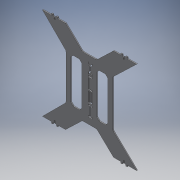
# Autodesk Inventor part: Z stage_brace
Saved by Autodesk Inventor 2019 (Build 230136000, 136)
## iProperties
Created: 2020-03-07
Part Number: Z stage_brace
Material: Generic
Document SubType Name: Modeling
Designer: Vijay
Density: 1 g/cm^3
Appearance: Default
Author: Vijay
Autodesk Inventor part; units mm, degrees
(part 1 of 2)
ref_plane "YZ Plane" through (0, 0, 0) normal (1, 0, 0) x (0, 1, 0)
ref_plane "XZ Plane" through (0, 0, 0) normal (0, 1, 0) x (-1, 0, 0)
ref_plane "XY Plane" through (0, 0, 0) normal (0, 0, 1) x (1, 0, 0)
sketch "Sketch1" plane through (0, 0, 0) normal (0, 0, 1) x (1, 0, 0)
  line L0 (428.582494, 0) -> (19.999963, 0)
  line L1 (19.999963, -400) -> (428.582494, -400)
  line L2 (328.588324, 0) -> (224.296824, -100)
  line L3 (224.296824, -100) -> (119.999963, 0)
  line L4 (328.582494, -400) -> (224.296824, -300)
  line L5 (224.296824, -300) -> (119.999963, -400)
  line L6 (224.296824, 24.036102) -> (224.296824, -493.226766) construction
  line L7 (428.582494, 0) -> (328.588324, 0)
  line L8 (119.999963, 0) -> (19.998423, 0)
  line L9 (19.999963, -400) -> (119.999963, -400)
  line L10 (328.582494, -400) -> (428.582446, -400)
  line L11 (19.998423, 0) -> (122.169678, -102.170786)
  line L12 (122.169678, -102.170786) -> (122.17075, -297.828745)
  line L13 (122.17075, -297.828745) -> (19.999963, -400)
  line L14 (428.582494, 0) -> (324.296824, -100.006079)
  line L15 (324.296824, -100.006079) -> (324.296824, -299.999951)
  line L16 (324.296824, -299.999951) -> (428.582446, -400)
  line L17 (255.584274, -70) -> (193.007766, -70)
  line L18 (255.582525, -330) -> (193.007766, -330)
  line L19 (19.999963, -400) -> (19.999963, -400)
  point P0 (0, 0)
  dimension "d1" = 100
  dimension "d2" = 100
  dimension "d3" = 100
  dimension "d4" = 104.2915
  dimension "d5" = 100
  dimension "d6" = 100
  dimension "d7" = 100
  dimension "d8" = 70
  dimension "d9" = 70
  constraints: 36 end point, 7 point on line, 4 equal length, 4 horizontal, 4 parallel, 3 perpendicular, 2 collinear, 2 vertical
  measures "d1" distance of L4.start L1.end
  measures "d2" distance of L5.end L1.start
  measures "d3" distance of L3.end L0.end
  measures "d4" distance from line of L6 L2.start
  measures "d5" distance from line of L0 L2.end
  measures "d6" distance from line of L1 L4.end
  measures "d7" distance between parallel lines of L6 L15
  measures "d8" distance between parallel lines of L0 L17
  measures "d9" distance between parallel lines of L1 L18
extrude "Extrusion1" add sketch "Sketch1" against normal blind 4 contours L14 L15 L16 L1 L4 L5 L13 L12 L11 L0 L3 L2 | L2 L3 L17 | L18 L5 L4
fillet "Fillet1" radius 10 8 edges at (324.2968, -100.0061, -2) (324.2968, -300, -2) (255.5825, -330, -2) (193.0078, -330, -2) (122.1708, -297.8287, -2) (122.1697, -102.1708, -2) (193.0078, -70, -2) (255.5843, -70, -2)
sketch "Sketch2" plane through (0, 0, -4) normal (0, 0, -1) x (-1, 0, 0)
  line L0 (-235.522226, -304.84913) -> (-235.522226, -94.876812) construction
  line L1 (-235.522226, -94.876812) -> (-217.757001, -94.876812) construction
  line L2 (-217.757001, -94.876812) -> (-217.757001, -304.84913) construction
  line L3 (-217.757001, -304.84913) -> (-235.522226, -304.84913) construction
  line L4 (-217.757, -297.116395) -> (-224.424748, -297.116395)
  line L5 (-224.424748, -297.116395) -> (-224.424748, -260.814212)
  line L6 (-224.424748, -260.814212) -> (-217.757, -260.814212)
  line L7 (-217.757, -260.814212) -> (-217.757, -255.057105)
  line L8 (-217.757, -255.057105) -> (-235.522226, -255.057105)
  line L9 (-235.522226, -255.057105) -> (-235.522226, -260.814212)
  line L10 (-235.522226, -260.814212) -> (-228.854478, -260.814212)
  line L11 (-228.854478, -260.814212) -> (-228.854478, -297.116395)
  line L12 (-228.854478, -297.116395) -> (-235.522226, -297.116395)
  line L13 (-235.522226, -297.116395) -> (-235.522226, -302.873501)
  line L14 (-235.522226, -302.873501) -> (-217.757, -302.873501)
  line L15 (-217.757, -302.873501) -> (-217.757, -297.116395)
  line L16 (-224.424748, -205.542904) -> (-228.854478, -205.542904)
  line L17 (-228.854478, -205.542904) -> (-228.854478, -245.348741)
  line L18 (-228.854478, -245.348741) -> (-229.76512, -245.348741)
  spline S0 degree 2 poles (-229.76512, -245.348741) (-230.305331, -245.348741) (-231.10793, -244.777661) (-231.10793, -244.160277) knots 0 0 0 1 2 2 2
  line L19 (-231.10793, -244.160277) -> (-231.10793, -205.4966)
  line L20 (-231.10793, -205.4966) -> (-235.522226, -205.4966)
  line L21 (-235.522226, -205.4966) -> (-235.522226, -247.170024)
  spline S1 degree 2 poles (-235.522226, -247.170024) (-235.522226, -249.238261) (-233.392251, -251.105847) (-231.555534, -251.105847) knots 0 0 0 1 2 2 2
  line L22 (-231.555534, -251.105847) -> (-221.723692, -251.105847)
  spline S2 degree 2 poles (-221.723692, -251.105847) (-219.886975, -251.105847) (-217.757, -249.238261) (-217.757, -247.170024) knots 0 0 0 1 2 2 2
  line L23 (-217.757, -247.170024) -> (-217.757, -205.4966)
  line L24 (-217.757, -205.4966) -> (-222.18673, -205.4966)
  line L25 (-222.18673, -205.4966) -> (-222.18673, -244.160277)
  spline S3 degree 2 poles (-222.18673, -244.160277) (-222.18673, -244.777661) (-222.973895, -245.348741) (-223.514106, -245.348741) knots 0 0 0 1 2 2 2
  line L26 (-223.514106, -245.348741) -> (-224.424748, -245.348741)
  line L27 (-224.424748, -245.348741) -> (-224.424748, -205.542904)
  line L28 (-235.522226, -201.545342) -> (-221.723692, -201.545342)
  spline S4 degree 2 poles (-221.723692, -201.545342) (-219.886975, -201.545342) (-217.757, -199.677755) (-217.757, -197.609519) knots 0 0 0 1 2 2 2
  line L29 (-217.757, -197.609519) -> (-217.757, -155.936094)
  line L30 (-217.757, -155.936094) -> (-222.18673, -155.936094)
  line L31 (-222.18673, -155.936094) -> (-222.18673, -194.599771)
  spline S5 degree 2 poles (-222.18673, -194.599771) (-222.18673, -195.217155) (-222.973895, -195.788236) (-223.514106, -195.788236) knots 0 0 0 1 2 2 2
  line L32 (-223.514106, -195.788236) -> (-235.522226, -195.788236)
  line L33 (-235.522226, -195.788236) -> (-235.522226, -201.545342)
  line L34 (-217.757, -146.181426) -> (-235.522226, -146.181426)
  line L35 (-235.522226, -146.181426) -> (-235.522226, -151.984836)
  line L36 (-235.522226, -151.984836) -> (-217.757, -151.984836)
  line L37 (-217.757, -151.984836) -> (-217.757, -146.181426)
  line L38 (-235.522226, -95.710279) -> (-235.522226, -103.304103)
  line L39 (-235.522226, -103.304103) -> (-228.854478, -111.422704)
  line L40 (-228.854478, -111.422704) -> (-228.854478, -127.659904)
  line L41 (-228.854478, -127.659904) -> (-235.522226, -135.778505)
  line L42 (-235.522226, -135.778505) -> (-235.522226, -143.372329)
  line L43 (-235.522226, -143.372329) -> (-226.64733, -132.768757)
  line L44 (-226.64733, -132.768757) -> (-217.757, -143.372329)
  line L45 (-217.757, -143.372329) -> (-217.757, -135.778505)
  line L46 (-217.757, -135.778505) -> (-224.424748, -127.659904)
  line L47 (-224.424748, -127.659904) -> (-224.424748, -111.422704)
  line L48 (-224.424748, -111.422704) -> (-217.757, -103.304103)
  line L49 (-217.757, -103.304103) -> (-217.757, -95.710279)
  line L50 (-217.757, -95.710279) -> (-226.64733, -106.31385)
  line L51 (-226.64733, -106.31385) -> (-235.522226, -95.710279)
  point P0 (0, 0)
  constraints: 2 other
extrude "Extrusion2" cut sketch "Sketch2" against normal blind 25.4
sketch "Sketch3" plane through (0, 0, 0) normal (0, 0, 1) x (1, 0, 0)
  line L0 (394.29103, -17.648783) -> (394.29103, 0)
  line L1 (394.29103, 0) -> (387.415198, 0)
  line L2 (387.415198, 0) -> (387.415198, 6.35)
  line L3 (387.415198, 6.35) -> (381.415186, 6.35)
  line L4 (381.415186, 6.35) -> (381.415186, 0)
  line L5 (381.415186, 0) -> (375.315187, 0)
  line L6 (375.315187, 0) -> (375.315187, -6)
  line L7 (375.315187, -6) -> (376.565186, -6)
  line L8 (376.565186, -6) -> (376.565186, -8)
  line L9 (376.565186, -8) -> (375.315187, -8)
  line L10 (375.315187, -8) -> (375.315187, -10.649999)
  line L11 (375.315187, -10.649999) -> (372.315196, -10.649999)
  line L12 (372.315196, -10.649999) -> (372.315196, -8)
  line L13 (372.315196, -8) -> (371.065197, -8)
  line L14 (371.065197, -8) -> (371.065197, -6)
  line L15 (371.065197, -6) -> (372.315196, -6)
  line L16 (372.315196, -6) -> (372.315196, 0)
  line L17 (372.315196, 0) -> (366.215197, 0)
  line L18 (366.215197, 0) -> (366.215197, 6.35)
  line L19 (366.215197, 6.35) -> (360.2152, 6.35)
  line L20 (360.2152, 6.35) -> (360.2152, 0)
  line L21 (360.2152, 0) -> (353.339353, 0)
  line L22 (353.339353, 0) -> (353.339353, -17.648783)
  line L23 (353.339353, -17.648783) -> (394.29103, -17.648783)
  line L24 (353.340387, -382.350485) -> (353.340487, -399.999268)
  line L25 (353.340487, -399.999268) -> (360.216319, -399.999229)
  line L26 (360.216319, -399.999229) -> (360.216355, -406.349229)
  line L27 (360.216355, -406.349229) -> (366.216367, -406.349195)
  line L28 (366.216367, -406.349195) -> (366.216331, -399.999195)
  line L29 (366.216331, -399.999195) -> (372.31633, -399.999161)
  line L30 (372.31633, -399.999161) -> (372.316296, -393.999161)
  line L31 (372.316296, -393.999161) -> (371.066297, -393.999168)
  line L32 (371.066297, -393.999168) -> (371.066286, -391.999167)
  line L33 (371.066286, -391.999167) -> (372.316284, -391.99916)
  line L34 (372.316284, -391.99916) -> (372.316269, -389.349161)
  line L35 (372.316269, -389.349161) -> (375.316261, -389.349144)
  line L36 (375.316261, -389.349144) -> (375.316276, -391.999143)
  line L37 (375.316276, -391.999143) -> (376.566274, -391.999136)
  line L38 (376.566274, -391.999136) -> (376.566286, -393.999137)
  line L39 (376.566286, -393.999137) -> (375.316287, -393.999144)
  line L40 (375.316287, -393.999144) -> (375.316321, -399.999144)
  line L41 (375.316321, -399.999144) -> (381.41632, -399.999109)
  line L42 (381.41632, -399.999109) -> (381.416356, -406.349109)
  line L43 (381.416356, -406.349109) -> (387.416353, -406.349075)
  line L44 (387.416353, -406.349075) -> (387.416317, -399.999075)
  line L45 (387.416317, -399.999075) -> (394.292164, -399.999036)
  line L46 (394.292164, -399.999036) -> (394.292064, -382.350253)
  line L47 (394.292064, -382.350253) -> (353.340387, -382.350485)
  line L48 (93.121147, -17.649526) -> (93.121047, -0.000743)
  line L49 (93.121047, -0.000743) -> (86.245215, -0.000782)
  line L50 (86.245215, -0.000782) -> (86.245179, 6.349218)
  line L51 (86.245179, 6.349218) -> (80.245166, 6.349184)
  line L52 (80.245166, 6.349184) -> (80.245202, -0.000816)
  line L53 (80.245202, -0.000816) -> (74.145203, -0.000851)
  line L54 (74.145203, -0.000851) -> (74.145237, -6.000851)
  line L55 (74.145237, -6.000851) -> (75.395236, -6.000844)
  line L56 (75.395236, -6.000844) -> (75.395248, -8.000844)
  line L57 (75.395248, -8.000844) -> (74.145249, -8.000851)
  line L58 (74.145249, -8.000851) -> (74.145264, -10.65085)
  line L59 (74.145264, -10.65085) -> (71.145273, -10.650867)
  line L60 (71.145273, -10.650867) -> (71.145258, -8.000868)
  line L61 (71.145258, -8.000868) -> (69.895259, -8.000875)
  line L62 (69.895259, -8.000875) -> (69.895247, -6.000875)
  line L63 (69.895247, -6.000875) -> (71.145246, -6.000868)
  line L64 (71.145246, -6.000868) -> (71.145212, -0.000868)
  line L65 (71.145212, -0.000868) -> (65.045213, -0.000902)
  line L66 (65.045213, -0.000902) -> (65.045177, 6.349097)
  line L67 (65.045177, 6.349097) -> (59.04518, 6.349063)
  line L68 (59.04518, 6.349063) -> (59.045216, -0.000936)
  line L69 (59.045216, -0.000936) -> (52.169369, -0.000975)
  line L70 (52.169369, -0.000975) -> (52.169469, -17.649759)
  line L71 (52.169469, -17.649759) -> (93.121147, -17.649526)
  line L72 (52.171537, -382.352192) -> (52.171637, -400.000976)
  line L73 (52.171637, -400.000976) -> (59.047469, -400.000937)
  line L74 (59.047469, -400.000937) -> (59.047505, -406.350936)
  line L75 (59.047505, -406.350936) -> (65.047517, -406.350902)
  line L76 (65.047517, -406.350902) -> (65.047481, -400.000903)
  line L77 (65.047481, -400.000903) -> (71.14748, -400.000868)
  line L78 (71.14748, -400.000868) -> (71.147446, -394.000868)
  line L79 (71.147446, -394.000868) -> (69.897447, -394.000875)
  line L80 (69.897447, -394.000875) -> (69.897436, -392.000875)
  line L81 (69.897436, -392.000875) -> (71.147434, -392.000868)
  line L82 (71.147434, -392.000868) -> (71.147419, -389.350868)
  line L83 (71.147419, -389.350868) -> (74.14741, -389.350851)
  line L84 (74.14741, -389.350851) -> (74.147426, -392.000851)
  line L85 (74.147426, -392.000851) -> (75.397424, -392.000843)
  line L86 (75.397424, -392.000843) -> (75.397436, -394.000844)
  line L87 (75.397436, -394.000844) -> (74.147437, -394.000851)
  line L88 (74.147437, -394.000851) -> (74.147471, -400.000851)
  line L89 (74.147471, -400.000851) -> (80.24747, -400.000816)
  line L90 (80.24747, -400.000816) -> (80.247506, -406.350816)
  line L91 (80.247506, -406.350816) -> (86.247503, -406.350782)
  line L92 (86.247503, -406.350782) -> (86.247467, -400.000782)
  line L93 (86.247467, -400.000782) -> (93.123314, -400.000743)
  line L94 (93.123314, -400.000743) -> (93.123214, -382.35196)
  line L95 (93.123214, -382.35196) -> (52.171537, -382.352192)
  point P0 (0, 0)
extrude "Extrusion3" add sketch "Sketch3" against normal up to surface (4 mm away)
sketch "Sketch4" plane through (0, 0, 0) normal (0, 0, 1) x (1, 0, 0)
  line L0 (394.29103, -17.648783) -> (394.29103, 0)
  line L1 (394.29103, 0) -> (387.415198, 0)
  line L2 (387.415198, 0) -> (387.415198, 6.35)
  line L3 (387.415198, 6.35) -> (381.415186, 6.35)
  line L4 (381.415186, 6.35) -> (381.415186, 0)
  line L5 (381.415186, 0) -> (375.315187, 0)
  line L6 (375.315187, 0) -> (375.315187, -6)
  line L7 (375.315187, -6) -> (376.565186, -6)
  line L8 (376.565186, -6) -> (376.565186, -8)
  line L9 (376.565186, -8) -> (375.315187, -8)
  line L10 (375.315187, -8) -> (375.315187, -10.649999)
  line L11 (375.315187, -10.649999) -> (372.315196, -10.649999)
  line L12 (372.315196, -10.649999) -> (372.315196, -8)
  line L13 (372.315196, -8) -> (371.065197, -8)
  line L14 (371.065197, -8) -> (371.065197, -6)
  line L15 (371.065197, -6) -> (372.315196, -6)
  line L16 (372.315196, -6) -> (372.315196, 0)
  line L17 (372.315196, 0) -> (366.215197, 0)
  line L18 (366.215197, 0) -> (366.215197, 6.35)
  line L19 (366.215197, 6.35) -> (360.2152, 6.35)
  line L20 (360.2152, 6.35) -> (360.2152, 0)
  line L21 (360.2152, 0) -> (353.339353, 0)
  line L22 (353.339353, 0) -> (353.339353, -17.648783)
  line L23 (353.339353, -17.648783) -> (394.29103, -17.648783)
  line L24 (353.340387, -382.350485) -> (353.340487, -399.999268)
  line L25 (353.340487, -399.999268) -> (360.216319, -399.999229)
  line L26 (360.216319, -399.999229) -> (360.216355, -406.349229)
  line L27 (360.216355, -406.349229) -> (366.216367, -406.349195)
  line L28 (366.216367, -406.349195) -> (366.216331, -400)
  line L29 (366.216331, -399.999195) -> (372.31633, -399.999161)
  line L30 (372.31633, -399.999161) -> (372.316296, -393.999161)
  line L31 (372.316296, -393.999161) -> (371.066297, -393.999168)
  line L32 (371.066297, -393.999168) -> (371.066286, -391.999167)
  line L33 (371.066286, -391.999167) -> (372.316284, -391.99916)
  line L34 (372.316284, -391.99916) -> (372.316269, -389.349161)
  line L35 (372.316269, -389.349161) -> (375.316261, -389.349144)
  line L36 (375.316261, -389.349144) -> (375.316276, -391.999143)
  line L37 (375.316276, -391.999143) -> (376.566274, -391.999136)
  line L38 (376.566274, -391.999136) -> (376.566286, -393.999137)
  line L39 (376.566286, -393.999137) -> (375.316287, -393.999144)
  line L40 (375.316287, -393.999144) -> (375.316321, -399.999144)
  line L41 (375.316321, -399.999144) -> (381.41632, -399.999109)
  line L42 (381.41632, -400) -> (381.416356, -406.349109)
  line L43 (381.416356, -406.349109) -> (387.416353, -406.349075)
  line L44 (387.416353, -406.349075) -> (387.416317, -399.999075)
  line L45 (387.416317, -399.999075) -> (394.292164, -399.999036)
  line L46 (394.292164, -399.999036) -> (394.292064, -382.350253)
  line L47 (394.292064, -382.350253) -> (353.340387, -382.350485)
  line L48 (52.171537, -382.352192) -> (52.171637, -400.000976)
  line L49 (52.171637, -400.000976) -> (59.047469, -400.000937)
  line L50 (59.047469, -400.000937) -> (59.047505, -406.350936)
  line L51 (59.047505, -406.350936) -> (65.047517, -406.350902)
  line L52 (65.047517, -406.350902) -> (65.047481, -400.000159)
  line L53 (93.123314, -400.000743) -> (71.14748, -400.000868)
  line L54 (71.14748, -400.000868) -> (71.147446, -394.000868)
  line L55 (71.147446, -394.000868) -> (69.897447, -394.000875)
  line L56 (69.897447, -394.000875) -> (69.897436, -392.000875)
  line L57 (69.897436, -392.000875) -> (71.147434, -392.000868)
  line L58 (71.147434, -392.000868) -> (71.147419, -389.350868)
  line L59 (71.147419, -389.350868) -> (74.14741, -389.350851)
  line L60 (74.14741, -389.350851) -> (74.147426, -392.000851)
  line L61 (74.147426, -392.000851) -> (75.397424, -392.000843)
  line L62 (75.397424, -392.000843) -> (75.397436, -394.000844)
  line L63 (75.397436, -394.000844) -> (74.147437, -394.000851)
  line L64 (74.147437, -394.000851) -> (74.147471, -400.000851)
  line L65 (74.147471, -400.000851) -> (119.999963, -400.000591)
  line L66 (80.24747, -400.000225) -> (80.247506, -406.350816)
  line L67 (80.247506, -406.350816) -> (86.247503, -406.350782)
  line L68 (86.247503, -406.350782) -> (86.247467, -400.000782)
  line L69 (86.247467, -400.000782) -> (93.123314, -400.000743)
  line L70 (93.123314, -400.000743) -> (93.123214, -382.35196)
  line L71 (93.123214, -382.35196) -> (52.171537, -382.352192)
  line L72 (93.121147, -17.649526) -> (93.121047, -0.000743)
  line L73 (93.121047, -0.000743) -> (86.245215, -0.000782)
  line L74 (86.245215, -0.000782) -> (86.245179, 6.349218)
  line L75 (86.245179, 6.349218) -> (80.245166, 6.349184)
  line L76 (80.245166, 6.349184) -> (80.245202, 0)
  line L77 (80.245202, -0.000816) -> (74.145203, -0.000851)
  line L78 (74.145203, -0.000851) -> (74.145237, -6.000851)
  line L79 (74.145237, -6.000851) -> (75.395236, -6.000844)
  line L80 (75.395236, -6.000844) -> (75.395248, -8.000844)
  line L81 (75.395248, -8.000844) -> (74.145249, -8.000851)
  line L82 (74.145249, -8.000851) -> (74.145264, -10.65085)
  line L83 (74.145264, -10.65085) -> (71.145273, -10.650867)
  line L84 (71.145273, -10.650867) -> (71.145258, -8.000868)
  line L85 (71.145258, -8.000868) -> (69.895259, -8.000875)
  line L86 (69.895259, -8.000875) -> (69.895247, -6.000875)
  line L87 (69.895247, -6.000875) -> (71.145246, -6.000868)
  line L88 (71.145246, -6.000868) -> (71.145212, -0.000868)
  line L89 (71.145212, -0.000868) -> (65.045213, -0.000902)
  line L90 (65.045213, 0) -> (65.045177, 6.349097)
  line L91 (65.045177, 6.349097) -> (59.04518, 6.349063)
  line L92 (59.04518, 6.349063) -> (59.045216, -0.000936)
  line L93 (59.045216, -0.000936) -> (52.169369, -0.000975)
  line L94 (52.169369, -0.000975) -> (52.169469, -17.649759)
  line L95 (52.169469, -17.649759) -> (93.121147, -17.649526)
  line L96 (375.315187, 0) -> (372.315196, 0)
  line L97 (375.316321, -400) -> (372.31633, -400)
  line L98 (366.216331, -400) -> (381.41632, -400)
  line L99 (74.147471, -400) -> (71.14748, -400)
  line L100 (119.999963, -400) -> (93.123314, -400)
  line L101 (74.145203, 0) -> (71.145212, 0)
  line L102 (65.045213, 0) -> (80.245202, 0)
  point P0 (0, 0)
  point P1 (93.123314, -400)
  point P2 (119.999963, -400)
  constraints: 8 end point, 3 horizontal, 1 perpendicular, 3 other
extrude "Extrusion4" cut sketch "Sketch4" against normal blind 25.4 contours L6 L7 L8 L9 L10 L11 L12 L13 L14 L15 L16 L96 | L30 L31 L32 L33 L34 L35 L36 L37 L38 L39 L40 L97 | L53 L54 L55 L56 L57 L58 L59 L60 L61 L62 L63 L64 | L78 L79 L80 L81 L82 L83 L84 L85 L86 L87 L88 L101
sketch "Sketch5" plane through (0, 0, -4) normal (0, 0, -1) x (-1, 0, 0)
  line L0 (-228.854478, -111.422704) -> (-235.522226, -103.304103)
  line L1 (-235.522226, -103.304103) -> (-235.522226, -95.710279)
  line L2 (-235.522226, -95.710279) -> (-226.64733, -106.31385)
  line L3 (-226.64733, -106.31385) -> (-217.757, -95.710279)
  line L4 (-217.757, -95.710279) -> (-217.757, -103.304103)
  line L5 (-217.757, -103.304103) -> (-224.424748, -111.422704)
  line L6 (-224.424748, -111.422704) -> (-224.424748, -127.659904)
  line L7 (-224.424748, -127.659904) -> (-217.757, -135.778505)
  line L8 (-217.757, -135.778505) -> (-217.757, -143.372329)
  line L9 (-217.757, -143.372329) -> (-226.64733, -132.768757)
  line L10 (-226.64733, -132.768757) -> (-235.522226, -143.372329)
  line L11 (-235.522226, -143.372329) -> (-235.522226, -135.778505)
  line L12 (-235.522226, -135.778505) -> (-228.854478, -127.659904)
  line L13 (-228.854478, -127.659904) -> (-228.854478, -111.422704)
  line L14 (-221.723692, -201.545342) -> (-235.522226, -201.545342)
  line L15 (-235.522226, -201.545342) -> (-235.522226, -195.788236)
  line L16 (-235.522226, -195.788236) -> (-223.514106, -195.788236)
  line L17 (-222.18673, -194.599771) -> (-222.18673, -155.936094)
  line L18 (-222.18673, -155.936094) -> (-217.757, -155.936094)
  line L19 (-217.757, -155.936094) -> (-217.757, -197.609519)
  line L20 (-224.424748, -260.814212) -> (-224.424748, -297.116395)
  line L21 (-224.424748, -297.116395) -> (-217.757, -297.116395)
  line L22 (-217.757, -297.116395) -> (-217.757, -302.873501)
  line L23 (-217.757, -302.873501) -> (-235.522226, -302.873501)
  line L24 (-235.522226, -302.873501) -> (-235.522226, -297.116395)
  line L25 (-235.522226, -297.116395) -> (-228.854478, -297.116395)
  line L26 (-228.854478, -297.116395) -> (-228.854478, -260.814212)
  line L27 (-228.854478, -260.814212) -> (-235.522226, -260.814212)
  line L28 (-235.522226, -260.814212) -> (-235.522226, -255.057105)
  line L29 (-235.522226, -255.057105) -> (-217.757, -255.057105)
  line L30 (-217.757, -255.057105) -> (-217.757, -260.814212)
  line L31 (-217.757, -260.814212) -> (-224.424748, -260.814212)
  line L32 (-228.854478, -245.348741) -> (-228.854478, -205.542904)
  line L33 (-228.854478, -205.542904) -> (-224.424748, -205.542904)
  line L34 (-224.424748, -205.542904) -> (-224.424748, -245.348741)
  line L35 (-224.424748, -245.348741) -> (-223.514106, -245.348741)
  line L36 (-222.18673, -244.160277) -> (-222.18673, -205.4966)
  line L37 (-222.18673, -205.4966) -> (-217.757, -205.4966)
  line L38 (-217.757, -205.4966) -> (-217.757, -247.170024)
  line L39 (-221.723692, -251.105847) -> (-231.555534, -251.105847)
  line L40 (-235.522226, -247.170024) -> (-235.522226, -205.4966)
  line L41 (-235.522226, -205.4966) -> (-231.10793, -205.4966)
  line L42 (-231.10793, -205.4966) -> (-231.10793, -244.160277)
  line L43 (-229.76512, -245.348741) -> (-228.854478, -245.348741)
  line L44 (-235.522226, -151.984836) -> (-235.522226, -146.181426)
  line L45 (-235.522226, -146.181426) -> (-217.757, -146.181426)
  line L46 (-217.757, -146.181426) -> (-217.757, -151.984836)
  line L47 (-217.757, -151.984836) -> (-235.522226, -151.984836)
  line L48 (-71.145212, -0.000868) -> (-71.145246, -6.000868)
  line L49 (-71.145246, -6.000868) -> (-69.895247, -6.000875)
  line L50 (-69.895247, -6.000875) -> (-69.895259, -8.000875)
  line L51 (-69.895259, -8.000875) -> (-71.145258, -8.000868)
  line L52 (-71.145258, -8.000868) -> (-71.145273, -10.650867)
  line L53 (-71.145273, -10.650867) -> (-74.145264, -10.65085)
  line L54 (-74.145264, -10.65085) -> (-74.145249, -8.000851)
  line L55 (-74.145249, -8.000851) -> (-75.395248, -8.000844)
  line L56 (-75.395248, -8.000844) -> (-75.395236, -6.000844)
  line L57 (-75.395236, -6.000844) -> (-74.145237, -6.000851)
  line L58 (-74.145237, -6.000851) -> (-74.145203, -0.000851)
  line L59 (-74.145203, -0.000851) -> (-71.145212, -0.000868)
  line L60 (-375.316321, -399.999144) -> (-375.316287, -393.999144)
  line L61 (-375.316287, -393.999144) -> (-376.566286, -393.999137)
  line L62 (-376.566286, -393.999137) -> (-376.566274, -391.999136)
  line L63 (-376.566274, -391.999136) -> (-375.316276, -391.999143)
  line L64 (-375.316276, -391.999143) -> (-375.316261, -389.349144)
  line L65 (-375.316261, -389.349144) -> (-372.316269, -389.349161)
  line L66 (-372.316269, -389.349161) -> (-372.316284, -391.99916)
  line L67 (-372.316284, -391.99916) -> (-371.066286, -391.999167)
  line L68 (-371.066286, -391.999167) -> (-371.066297, -393.999168)
  line L69 (-371.066297, -393.999168) -> (-372.316296, -393.999161)
  line L70 (-372.316296, -393.999161) -> (-372.31633, -399.999161)
  line L71 (-372.31633, -399.999161) -> (-375.316321, -399.999144)
  line L72 (-74.147471, -400.000851) -> (-74.147437, -394.000851)
  line L73 (-74.147437, -394.000851) -> (-75.397436, -394.000844)
  line L74 (-75.397436, -394.000844) -> (-75.397424, -392.000843)
  line L75 (-75.397424, -392.000843) -> (-74.147426, -392.000851)
  line L76 (-74.147426, -392.000851) -> (-74.14741, -389.350851)
  line L77 (-74.14741, -389.350851) -> (-71.147419, -389.350868)
  line L78 (-71.147419, -389.350868) -> (-71.147434, -392.000868)
  line L79 (-71.147434, -392.000868) -> (-69.897436, -392.000875)
  line L80 (-69.897436, -392.000875) -> (-69.897447, -394.000875)
  line L81 (-69.897447, -394.000875) -> (-71.147446, -394.000868)
  line L82 (-71.14748, -400.000868) -> (-71.147446, -394.000868)
  line L83 (-65.047481, -400.000903) -> (-71.14748, -400.000868)
  line L84 (-65.047517, -406.350902) -> (-65.047481, -400.000903)
  line L85 (-59.047505, -406.350936) -> (-65.047517, -406.350902)
  line L86 (-59.047469, -400.000937) -> (-59.047505, -406.350936)
  line L87 (-52.171637, -400.000976) -> (-59.047469, -400.000937)
  line L88 (-52.171637, -400) -> (-52.171637, -400.000976)
  line L89 (-52.171637, -400) -> (-19.999963, -400)
  line L90 (-19.999963, -400) -> (-119.241811, -300.757697)
  arc A0 (-122.170727, -293.68659) -> (-119.241811, -300.757697) centre (-112.170727, -293.686645) ccw
  line L91 (-122.170727, -293.68659) -> (-122.1697, -106.312903)
  arc A1 (-119.240752, -99.241874) -> (-122.1697, -106.312903) centre (-112.1697, -106.312958) ccw
  line L92 (-119.240752, -99.241874) -> (-19.998423, 0)
  line L93 (-19.998423, 0) -> (-59.045216, 0)
  line L94 (-59.04518, 6.349063) -> (-59.045216, 0)
  line L95 (-65.045177, 6.349097) -> (-59.04518, 6.349063)
  line L96 (-65.045213, 0) -> (-65.045177, 6.349097)
  line L97 (-65.045213, 0) -> (-80.245202, 0)
  line L98 (-80.245166, 6.349184) -> (-80.245202, 0)
  line L99 (-86.245179, 6.349218) -> (-80.245166, 6.349184)
  line L100 (-86.245215, 0) -> (-86.245179, 6.349218)
  line L101 (-86.245215, 0) -> (-119.999963, 0)
  line L102 (-119.999963, 0) -> (-190.106428, -67.218193)
  arc A2 (-197.027244, -70) -> (-190.106428, -67.218193) centre (-197.027244, -60) ccw
  line L103 (-197.027244, -70) -> (-251.564646, -70)
  arc A3 (-258.485647, -67.218015) -> (-251.564646, -70) centre (-251.564646, -60) ccw
  line L104 (-258.485647, -67.218015) -> (-328.588324, 0)
  line L105 (-328.588324, 0) -> (-360.2152, 0)
  line L106 (-360.2152, 6.35) -> (-360.2152, 0)
  line L107 (-366.215197, 6.35) -> (-360.2152, 6.35)
  line L108 (-366.215197, 0) -> (-366.215197, 6.35)
  line L109 (-366.215197, 0) -> (-372.315196, 0)
  line L110 (-372.315196, 0) -> (-372.315196, -6)
  line L111 (-372.315196, -6) -> (-371.065197, -6)
  line L112 (-371.065197, -6) -> (-371.065197, -8)
  line L113 (-371.065197, -8) -> (-372.315196, -8)
  line L114 (-372.315196, -8) -> (-372.315196, -10.649999)
  line L115 (-372.315196, -10.649999) -> (-375.315187, -10.649999)
  line L116 (-375.315187, -10.649999) -> (-375.315187, -8)
  line L117 (-375.315187, -8) -> (-376.565186, -8)
  line L118 (-376.565186, -8) -> (-376.565186, -6)
  line L119 (-376.565186, -6) -> (-375.315187, -6)
  line L120 (-375.315187, -6) -> (-375.315187, 0)
  line L121 (-375.315187, 0) -> (-381.415186, 0)
  line L122 (-381.415186, 6.35) -> (-381.415186, 0)
  line L123 (-387.415198, 6.35) -> (-381.415186, 6.35)
  line L124 (-387.415198, 0) -> (-387.415198, 6.35)
  line L125 (-387.415198, 0) -> (-428.582494, 0)
  line L126 (-428.582494, 0) -> (-327.375402, -97.053837)
  arc A4 (-324.296824, -104.271449) -> (-327.375402, -97.053837) centre (-334.296824, -104.271449) ccw
  line L127 (-324.296824, -104.271449) -> (-324.296824, -295.734404)
  arc A5 (-327.375618, -302.952223) -> (-324.296824, -295.734404) centre (-334.296824, -295.734404) ccw
  line L128 (-327.375618, -302.952223) -> (-428.582446, -400)
  line L129 (-428.582446, -400) -> (-387.416317, -400)
  line L130 (-387.416353, -406.349075) -> (-387.416317, -400)
  line L131 (-381.416356, -406.349109) -> (-387.416353, -406.349075)
  line L132 (-381.41632, -400) -> (-381.416356, -406.349109)
  line L133 (-381.41632, -400) -> (-366.216331, -400)
  line L134 (-366.216367, -406.349195) -> (-366.216331, -400)
  line L135 (-360.216355, -406.349229) -> (-366.216367, -406.349195)
  line L136 (-360.216319, -400) -> (-360.216355, -406.349229)
  line L137 (-360.216319, -400) -> (-328.582494, -400)
  line L138 (-328.582494, -400) -> (-258.483937, -332.782178)
  arc A6 (-251.562735, -330) -> (-258.483937, -332.782178) centre (-251.562735, -340) ccw
  line L139 (-251.562735, -330) -> (-197.027244, -330)
  arc A7 (-190.106428, -332.781807) -> (-197.027244, -330) centre (-197.027244, -340) ccw
  line L140 (-190.106428, -332.781807) -> (-119.999963, -400)
  line L141 (-119.999963, -400) -> (-93.123314, -400)
  line L142 (-93.123314, -400.000743) -> (-93.123314, -400)
  line L143 (-86.247467, -400.000782) -> (-93.123314, -400.000743)
  line L144 (-86.247503, -406.350782) -> (-86.247467, -400.000782)
  line L145 (-80.247506, -406.350816) -> (-86.247503, -406.350782)
  line L146 (-80.24747, -400.000816) -> (-80.247506, -406.350816)
  line L147 (-74.147471, -400.000851) -> (-80.24747, -400.000816)
  line L148 (-255.300194, -104.271449) -> (-304.296824, -104.271449)
  line L149 (-304.296824, -104.271449) -> (-304.296824, -295.734404)
  line L150 (-304.296824, -295.734404) -> (-255.300194, -295.734404)
  line L151 (-255.300194, -295.734404) -> (-255.300194, -104.271449)
  line L152 (-255.300194, -104.271449) -> (-304.296824, -295.734404) construction
  line L153 (-304.296824, -104.271449) -> (-255.300194, -295.734404) construction
  line L154 (-191.167357, -104.271449) -> (-142.170727, -104.271449)
  line L155 (-142.170727, -104.271449) -> (-142.170727, -295.734404)
  line L156 (-142.170727, -295.734404) -> (-191.167357, -295.734404)
  line L157 (-191.167357, -295.734404) -> (-191.167357, -104.271449)
  line L158 (-191.167357, -104.271449) -> (-142.170727, -295.734404) construction
  line L159 (-142.170727, -104.271449) -> (-191.167357, -295.734404) construction
  point P0 (0, 0)
  point P1 (-279.798509, -200.002927)
  point P2 (-166.669042, -200.002927)
  dimension "d19" = 20
  dimension "d20" = 20
  constraints: 24 end point, 4 midpoint, 4 parallel, 3 collinear, 2 horizontal, 2 perpendicular, 2 point on line, 6 other
  measures "d19" distance between parallel lines of L149 L127
  measures "d20" horizontal distance of L91.start L155.end
extrude "Extrusion5" cut sketch "Sketch5" against normal through all contours L151 L150 L149 L148 | L154 L155 L156 L157
chamfer "Chamfer1" distance 11.1125 angle 45 8 edges at (304.2968, -295.7344, -2) (255.3002, -295.7344, -2) (255.3002, -104.2714, -2) (304.2968, -104.2714, -2) (191.1674, -295.7344, -2) (142.1707, -295.7344, -2) (142.1707, -104.2714, -2) (191.1674, -104.2714, -2)
sketch "Sketch6" plane through (0, 0, 0) normal (0, 0, 1) x (1, 0, 0)
  line L0 (304.296824, -115.383949) -> (304.296824, -284.621904)
  line L1 (293.184324, -295.734404) -> (304.296824, -284.621904)
  line L2 (293.184324, -295.734404) -> (266.412694, -295.734404)
  line L3 (255.300194, -284.621904) -> (266.412694, -295.734404)
  line L4 (255.300194, -284.621904) -> (255.300194, -115.383949)
  line L5 (266.412694, -104.271449) -> (255.300194, -115.383949)
  line L6 (266.412694, -104.271449) -> (293.184324, -104.271449)
  line L7 (304.296824, -115.383949) -> (293.184324, -104.271449)
  line L8 (191.167357, -115.383949) -> (191.167357, -284.621904)
  line L9 (180.054857, -295.734404) -> (191.167357, -284.621904)
  line L10 (180.054857, -295.734404) -> (153.283227, -295.734404)
  line L11 (142.170727, -284.621904) -> (153.283227, -295.734404)
  line L12 (142.170727, -284.621904) -> (142.170727, -115.383949)
  line L13 (153.283227, -104.271449) -> (142.170727, -115.383949)
  line L14 (153.283227, -104.271449) -> (180.054857, -104.271449)
  line L15 (191.167357, -115.383949) -> (180.054857, -104.271449)
  line L16 (74.147437, -394.000851) -> (74.147471, -400.000851)
  line L17 (74.147471, -400.000851) -> (80.24747, -400.000816)
  line L18 (80.24747, -400.000816) -> (80.247506, -406.350816)
  line L19 (80.247506, -406.350816) -> (86.247503, -406.350782)
  line L20 (86.247503, -406.350782) -> (86.247467, -400.000782)
  line L21 (86.247467, -400.000782) -> (93.123314, -400.000743)
  line L22 (93.123314, -400.000743) -> (93.123314, -400)
  line L23 (93.123314, -400) -> (119.999963, -400)
  line L24 (119.999963, -400) -> (190.106428, -332.781807)
  arc A0 (197.027244, -330) -> (190.106428, -332.781807) centre (197.027244, -340) ccw
  line L25 (197.027244, -330) -> (251.562735, -330)
  arc A1 (258.483937, -332.782178) -> (251.562735, -330) centre (251.562735, -340) ccw
  line L26 (258.483937, -332.782178) -> (328.582494, -400)
  line L27 (328.582494, -400) -> (360.216319, -400)
  line L28 (360.216319, -400) -> (360.216355, -406.349229)
  line L29 (360.216355, -406.349229) -> (366.216367, -406.349195)
  line L30 (366.216367, -406.349195) -> (366.216331, -400)
  line L31 (366.216331, -400) -> (381.41632, -400)
  line L32 (381.41632, -400) -> (381.416356, -406.349109)
  line L33 (381.416356, -406.349109) -> (387.416353, -406.349075)
  line L34 (387.416353, -406.349075) -> (387.416317, -400)
  line L35 (387.416317, -400) -> (428.582446, -400)
  line L36 (428.582446, -400) -> (327.375618, -302.952223)
  arc A2 (324.296824, -295.734404) -> (327.375618, -302.952223) centre (334.296824, -295.734404) ccw
  line L37 (324.296824, -295.734404) -> (324.296824, -104.271449)
  arc A3 (327.375402, -97.053837) -> (324.296824, -104.271449) centre (334.296824, -104.271449) ccw
  line L38 (327.375402, -97.053837) -> (428.582494, 0)
  line L39 (428.582494, 0) -> (387.415198, 0)
  line L40 (387.415198, 0) -> (387.415198, 6.35)
  line L41 (387.415198, 6.35) -> (381.415186, 6.35)
  line L42 (381.415186, 6.35) -> (381.415186, 0)
  line L43 (381.415186, 0) -> (375.315187, 0)
  line L44 (375.315187, 0) -> (375.315187, -6)
  line L45 (375.315187, -6) -> (376.565186, -6)
  line L46 (376.565186, -6) -> (376.565186, -8)
  line L47 (376.565186, -8) -> (375.315187, -8)
  line L48 (375.315187, -8) -> (375.315187, -10.649999)
  line L49 (375.315187, -10.649999) -> (372.315196, -10.649999)
  line L50 (372.315196, -10.649999) -> (372.315196, -8)
  line L51 (372.315196, -8) -> (371.065197, -8)
  line L52 (371.065197, -8) -> (371.065197, -6)
  line L53 (371.065197, -6) -> (372.315196, -6)
  line L54 (372.315196, -6) -> (372.315196, 0)
  line L55 (372.315196, 0) -> (366.215197, 0)
  line L56 (366.215197, 0) -> (366.215197, 6.35)
  line L57 (366.215197, 6.35) -> (360.2152, 6.35)
  line L58 (360.2152, 6.35) -> (360.2152, 0)
  line L59 (360.2152, 0) -> (328.588324, 0)
  line L60 (328.588324, 0) -> (258.485647, -67.218015)
  arc A4 (251.564646, -70) -> (258.485647, -67.218015) centre (251.564646, -60) ccw
  line L61 (251.564646, -70) -> (197.027244, -70)
  arc A5 (190.106428, -67.218193) -> (197.027244, -70) centre (197.027244, -60) ccw
  line L62 (190.106428, -67.218193) -> (119.999963, 0)
  line L63 (119.999963, 0) -> (86.245215, 0)
  line L64 (86.245215, 0) -> (86.245179, 6.349218)
  line L65 (86.245179, 6.349218) -> (80.245166, 6.349184)
  line L66 (80.245166, 6.349184) -> (80.245202, 0)
  line L67 (80.245202, 0) -> (65.045213, 0)
  line L68 (65.045213, 0) -> (65.045177, 6.349097)
  line L69 (65.045177, 6.349097) -> (59.04518, 6.349063)
  line L70 (59.04518, 6.349063) -> (59.045216, 0)
  line L71 (59.045216, 0) -> (19.998423, 0)
  line L72 (19.998423, 0) -> (119.240752, -99.241874)
  arc A6 (122.1697, -106.312903) -> (119.240752, -99.241874) centre (112.1697, -106.312958) ccw
  line L73 (122.1697, -106.312903) -> (122.170727, -293.68659)
  arc A7 (119.241811, -300.757697) -> (122.170727, -293.68659) centre (112.170727, -293.686645) ccw
  line L74 (119.241811, -300.757697) -> (19.999963, -400)
  line L75 (19.999963, -400) -> (52.171637, -400)
  line L76 (52.171637, -400) -> (52.171637, -400.000976)
  line L77 (52.171637, -400.000976) -> (59.047469, -400.000937)
  line L78 (59.047469, -400.000937) -> (59.047505, -406.350936)
  line L79 (59.047505, -406.350936) -> (65.047517, -406.350902)
  line L80 (65.047517, -406.350902) -> (65.047481, -400.000903)
  line L81 (65.047481, -400.000903) -> (71.14748, -400.000868)
  line L82 (71.14748, -400.000868) -> (71.147446, -394.000868)
  line L83 (71.147446, -394.000868) -> (69.897447, -394.000875)
  line L84 (69.897447, -394.000875) -> (69.897436, -392.000875)
  line L85 (69.897436, -392.000875) -> (71.147434, -392.000868)
  line L86 (71.147434, -392.000868) -> (71.147419, -389.350868)
  line L87 (71.147419, -389.350868) -> (74.14741, -389.350851)
  line L88 (74.14741, -389.350851) -> (74.147426, -392.000851)
  line L89 (74.147426, -392.000851) -> (75.397424, -392.000843)
  line L90 (75.397424, -392.000843) -> (75.397436, -394.000844)
  line L91 (75.397436, -394.000844) -> (74.147437, -394.000851)
  line L92 (375.316287, -393.999144) -> (375.316321, -399.999144)
  line L93 (375.316321, -399.999144) -> (372.31633, -399.999161)
  line L94 (372.31633, -399.999161) -> (372.316296, -393.999161)
  line L95 (372.316296, -393.999161) -> (371.066297, -393.999168)
  line L96 (371.066297, -393.999168) -> (371.066286, -391.999167)
  line L97 (371.066286, -391.999167) -> (372.316284, -391.99916)
  line L98 (372.316284, -391.99916) -> (372.316269, -389.349161)
  line L99 (372.316269, -389.349161) -> (375.316261, -389.349144)
  line L100 (375.316261, -389.349144) -> (375.316276, -391.999143)
  line L101 (375.316276, -391.999143) -> (376.566274, -391.999136)
  line L102 (376.566274, -391.999136) -> (376.566286, -393.999137)
  line L103 (376.566286, -393.999137) -> (375.316287, -393.999144)
  line L104 (71.145246, -6.000868) -> (71.145212, -0.000868)
  line L105 (71.145212, -0.000868) -> (74.145203, -0.000851)
  line L106 (74.145203, -0.000851) -> (74.145237, -6.000851)
  line L107 (74.145237, -6.000851) -> (75.395236, -6.000844)
  line L108 (75.395236, -6.000844) -> (75.395248, -8.000844)
  line L109 (75.395248, -8.000844) -> (74.145249, -8.000851)
  line L110 (74.145249, -8.000851) -> (74.145264, -10.65085)
  line L111 (74.145264, -10.65085) -> (71.145273, -10.650867)
  line L112 (71.145273, -10.650867) -> (71.145258, -8.000868)
  line L113 (71.145258, -8.000868) -> (69.895259, -8.000875)
  line L114 (69.895259, -8.000875) -> (69.895247, -6.000875)
  line L115 (69.895247, -6.000875) -> (71.145246, -6.000868)
  line L116 (235.522226, -146.181426) -> (235.522226, -151.984836)
  line L117 (235.522226, -151.984836) -> (217.757, -151.984836)
  line L118 (217.757, -151.984836) -> (217.757, -146.181426)
  line L119 (217.757, -146.181426) -> (235.522226, -146.181426)
  line L120 (228.854478, -205.542904) -> (228.854478, -245.348741)
  line L121 (228.854478, -245.348741) -> (229.76512, -245.348741)
  line L122 (231.10793, -244.160277) -> (231.10793, -205.4966)
  line L123 (231.10793, -205.4966) -> (235.522226, -205.4966)
  line L124 (235.522226, -205.4966) -> (235.522226, -247.170024)
  line L125 (231.555534, -251.105847) -> (221.723692, -251.105847)
  line L126 (217.757, -247.170024) -> (217.757, -205.4966)
  line L127 (217.757, -205.4966) -> (222.18673, -205.4966)
  line L128 (222.18673, -205.4966) -> (222.18673, -244.160277)
  line L129 (223.514106, -245.348741) -> (224.424748, -245.348741)
  line L130 (224.424748, -245.348741) -> (224.424748, -205.542904)
  line L131 (224.424748, -205.542904) -> (228.854478, -205.542904)
  line L132 (224.424748, -297.116395) -> (224.424748, -260.814212)
  line L133 (224.424748, -260.814212) -> (217.757, -260.814212)
  line L134 (217.757, -260.814212) -> (217.757, -255.057105)
  line L135 (217.757, -255.057105) -> (235.522226, -255.057105)
  line L136 (235.522226, -255.057105) -> (235.522226, -260.814212)
  line L137 (235.522226, -260.814212) -> (228.854478, -260.814212)
  line L138 (228.854478, -260.814212) -> (228.854478, -297.116395)
  line L139 (228.854478, -297.116395) -> (235.522226, -297.116395)
  line L140 (235.522226, -297.116395) -> (235.522226, -302.873501)
  line L141 (235.522226, -302.873501) -> (217.757, -302.873501)
  line L142 (217.757, -302.873501) -> (217.757, -297.116395)
  line L143 (217.757, -297.116395) -> (224.424748, -297.116395)
  line L144 (217.757, -197.609519) -> (217.757, -155.936094)
  line L145 (217.757, -155.936094) -> (222.18673, -155.936094)
  line L146 (222.18673, -155.936094) -> (222.18673, -194.599771)
  line L147 (223.514106, -195.788236) -> (235.522226, -195.788236)
  line L148 (235.522226, -195.788236) -> (235.522226, -201.545342)
  line L149 (235.522226, -201.545342) -> (221.723692, -201.545342)
  line L150 (235.522226, -103.304103) -> (228.854478, -111.422704)
  line L151 (228.854478, -111.422704) -> (228.854478, -127.659904)
  line L152 (228.854478, -127.659904) -> (235.522226, -135.778505)
  line L153 (235.522226, -135.778505) -> (235.522226, -143.372329)
  line L154 (235.522226, -143.372329) -> (226.64733, -132.768757)
  line L155 (226.64733, -132.768757) -> (217.757, -143.372329)
  line L156 (217.757, -143.372329) -> (217.757, -135.778505)
  line L157 (217.757, -135.778505) -> (224.424748, -127.659904)
  line L158 (224.424748, -127.659904) -> (224.424748, -111.422704)
  line L159 (224.424748, -111.422704) -> (217.757, -103.304103)
  line L160 (217.757, -103.304103) -> (217.757, -95.710279)
  line L161 (217.757, -95.710279) -> (226.64733, -106.31385)
  line L162 (226.64733, -106.31385) -> (235.522226, -95.710279)
  line L163 (235.522226, -95.710279) -> (235.522226, -103.304103)
  line L164 (375.515187, -5.8) -> (375.515187, -0.2)
  line L165 (376.564053, -0.2) -> (381.615186, -0.2)
  line L166 (381.615186, -0.2) -> (381.615186, 6.15)
  line L167 (381.615186, 6.15) -> (387.215198, 6.15)
  line L168 (387.215198, 6.15) -> (387.215198, -0.2)
  line L169 (387.215198, -0.2) -> (428.084977, -0.2)
  line L170 (428.084977, -0.2) -> (327.236974, -96.909485)
  arc A8 (327.236974, -96.909485) -> (324.096824, -104.271449) centre (334.296824, -104.271449) ccw
  line L171 (324.096824, -104.271449) -> (324.096824, -295.734404)
  arc A9 (324.096824, -295.734404) -> (327.237194, -303.096579) centre (334.296824, -295.734404) ccw
  line L172 (327.237194, -303.096579) -> (428.084908, -399.8)
  line L173 (428.084908, -399.8) -> (387.216316, -399.8)
  line L174 (387.216316, -399.8) -> (387.216352, -406.149076)
  line L175 (387.216352, -406.149076) -> (381.616355, -406.149108)
  line L176 (381.616355, -406.149108) -> (381.616319, -399.8)
  line L177 (366.01633, -399.8) -> (366.016366, -406.149196)
  line L178 (366.016366, -406.149196) -> (360.416354, -406.149228)
  line L179 (360.416354, -406.149228) -> (360.416318, -399.8)
  line L180 (360.416318, -399.8) -> (328.66289, -399.8)
  line L181 (328.66289, -399.8) -> (258.622361, -332.637821)
  arc A10 (258.622361, -332.637821) -> (251.562735, -329.8) centre (251.562735, -340) ccw
  line L182 (251.562735, -329.8) -> (197.027244, -329.8)
  arc A11 (197.027244, -329.8) -> (189.968012, -332.637443) centre (197.027244, -340) ccw
  line L183 (189.968012, -332.637443) -> (119.919574, -399.8)
  line L184 (119.919574, -399.8) -> (92.923313, -399.8)
  line L185 (92.923313, -399.8) -> (92.923313, -399.800745)
  line L186 (92.923313, -399.800745) -> (86.047466, -399.800783)
  line L187 (86.047466, -399.800783) -> (86.047502, -406.150783)
  line L188 (86.047502, -406.150783) -> (80.447505, -406.150815)
  line L189 (80.447505, -406.150815) -> (80.447469, -399.800815)
  line L190 (80.447469, -399.800815) -> (75.397469, -399.800844)
  line L191 (74.34747, -399.80085) -> (74.347438, -394.20085)
  line L192 (74.347438, -394.20085) -> (75.597437, -394.200843)
  line L193 (75.597437, -394.200843) -> (75.597423, -391.800842)
  line L194 (75.597423, -391.800842) -> (74.347424, -391.800849)
  line L195 (74.347424, -391.800849) -> (74.347409, -389.15085)
  line L196 (74.347409, -389.15085) -> (70.947418, -389.150869)
  line L197 (70.947418, -389.150869) -> (70.947433, -391.800869)
  line L198 (70.947433, -391.800869) -> (69.697434, -391.800876)
  line L199 (69.697434, -391.800876) -> (69.697448, -394.200876)
  line L200 (69.697448, -394.200876) -> (70.947447, -394.200869)
  line L201 (70.947447, -394.200869) -> (70.947479, -399.800869)
  line L202 (69.89748, -399.800875) -> (64.84748, -399.800904)
  line L203 (64.84748, -399.800904) -> (64.847516, -406.150904)
  line L204 (64.847516, -406.150904) -> (59.247503, -406.150935)
  line L205 (59.247503, -406.150935) -> (59.247467, -399.800935)
  line L206 (59.247467, -399.800935) -> (52.371635, -399.800974)
  line L207 (52.371635, -399.800974) -> (52.371635, -399.8)
  line L208 (52.371635, -399.8) -> (20.482805, -399.8)
  line L209 (20.482805, -399.8) -> (119.383233, -300.899118)
  arc A12 (119.383233, -300.899118) -> (122.370727, -293.686589) centre (112.170727, -293.686645) ccw
  line L210 (122.370727, -293.686589) -> (122.3697, -106.312902)
  arc A13 (122.3697, -106.312902) -> (119.382173, -99.100453) centre (112.1697, -106.312958) ccw
  line L211 (119.382173, -99.100453) -> (20.481267, -0.2)
  line L212 (20.481267, -0.2) -> (59.245217, -0.2)
  line L213 (59.245217, -0.2) -> (59.245181, 6.149065)
  line L214 (59.245181, 6.149065) -> (64.845178, 6.149096)
  line L215 (64.845178, 6.149096) -> (64.845214, -0.2)
  line L216 (64.845214, -0.2) -> (80.445204, -0.2)
  line L217 (80.445204, -0.2) -> (80.445168, 6.149185)
  line L218 (80.445168, 6.149185) -> (86.04518, 6.149217)
  line L219 (86.04518, 6.149217) -> (86.045216, -0.2)
  line L220 (86.045216, -0.2) -> (119.919574, -0.2)
  line L221 (119.919574, -0.2) -> (189.968012, -67.362557)
  arc A14 (189.968012, -67.362557) -> (197.027244, -70.2) centre (197.027244, -60) ccw
  line L222 (197.027244, -70.2) -> (251.564646, -70.2)
  arc A15 (251.564646, -70.2) -> (258.624067, -67.362376) centre (251.564646, -60) ccw
  line L223 (258.624067, -67.362376) -> (328.668716, -0.2)
  line L224 (328.668716, -0.2) -> (360.4152, -0.2)
  line L225 (360.4152, -0.2) -> (360.4152, 6.15)
  line L226 (360.4152, 6.15) -> (366.015197, 6.15)
  line L227 (366.015197, 6.15) -> (366.015197, -0.2)
  line L228 (372.115196, -0.2) -> (372.115196, -5.8)
  line L229 (372.115196, -5.8) -> (370.865197, -5.8)
  line L230 (370.865197, -5.8) -> (370.865197, -8.2)
  line L231 (370.865197, -8.2) -> (372.115196, -8.2)
  line L232 (372.115196, -8.2) -> (372.115196, -10.849999)
  line L233 (372.115196, -10.849999) -> (375.515187, -10.849999)
  line L234 (375.515187, -10.849999) -> (375.515187, -8.2)
  line L235 (375.515187, -8.2) -> (376.765186, -8.2)
  line L236 (376.765186, -8.2) -> (376.765186, -5.8)
  line L237 (376.765186, -5.8) -> (375.515187, -5.8)
  line L238 (375.515187, -0.2) -> (375.515187, 0)
  line L239 (375.315187, 0) -> (381.415186, 0)
  line L240 (372.115196, -0.2) -> (372.115196, 0)
  line L241 (366.215197, 0) -> (372.315196, 0)
  line L242 (375.516274, -391.799142) -> (375.516259, -389.149143)
  line L243 (375.516259, -389.149143) -> (372.116268, -389.149162)
  line L244 (372.116268, -389.149162) -> (372.116283, -391.799161)
  line L245 (372.116283, -391.799161) -> (370.866284, -391.799169)
  line L246 (370.866284, -391.799169) -> (370.866298, -394.199169)
  line L247 (370.866298, -394.199169) -> (372.116297, -394.199162)
  line L248 (372.116297, -394.199162) -> (372.116331, -400.199162)
  line L249 (372.116331, -400.199162) -> (375.516322, -400.199143)
  line L250 (375.516322, -400.199143) -> (375.516288, -394.199143)
  line L251 (375.516288, -394.199143) -> (376.766287, -394.199135)
  line L252 (376.766287, -394.199135) -> (376.766273, -391.799135)
  line L253 (376.766273, -391.799135) -> (375.516274, -391.799142)
  line L254 (74.345236, -5.80085) -> (74.345202, 0.19915)
  line L255 (74.345202, 0.19915) -> (70.945211, 0.199131)
  line L256 (70.945211, 0.199131) -> (70.945245, -5.800869)
  line L257 (70.945245, -5.800869) -> (69.695246, -5.800876)
  line L258 (69.695246, -5.800876) -> (69.69526, -8.200876)
  line L259 (69.69526, -8.200876) -> (70.945259, -8.200869)
  line L260 (70.945259, -8.200869) -> (70.945274, -10.850869)
  line L261 (70.945274, -10.850869) -> (74.345265, -10.850849)
  line L262 (74.345265, -10.850849) -> (74.34525, -8.20085)
  line L263 (74.34525, -8.20085) -> (75.595249, -8.200843)
  line L264 (75.595249, -8.200843) -> (75.595235, -5.800843)
  line L265 (75.595235, -5.800843) -> (74.345236, -5.80085)
  line L266 (74.34747, -399.80085) -> (74.347471, -400.00085)
  line L267 (74.147471, -400.000851) -> (80.24747, -400.000816)
  line L268 (70.947479, -399.800869) -> (70.94748, -400.000869)
  line L269 (65.047481, -400.000903) -> (71.14748, -400.000868)
  line L270 (366.015197, -0.2) -> (371.065197, -0.2)
  line L271 (372.114063, -0.2) -> (372.115196, -0.2)
  line L272 (372.116329, -399.8) -> (372.115196, -399.8)
  line L273 (371.06633, -399.8) -> (366.01633, -399.8)
  point P0 (0, 0)
  dimension "d2" = 100
  dimension "d26" = 0.2
  dimension "d27" = 0.2
  dimension "d28" = 0.2
  constraints: 212 end point, 16 point on circle, 12 point on line, 8 centre point, 2 parallel, 2 perpendicular, 101 other
  measures "d26" distance between parallel lines of L44 L164
  measures "d27" distance between parallel lines of L100 L242
  measures "d28" distance between parallel lines of L106 L254